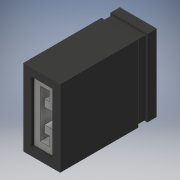
# Autodesk Inventor part: Jumper
Saved by Autodesk Inventor 2017 SP1 (Build 210196100, 196)
## iProperties
Part Number: Jumper
Material: Generisch
Document SubType Name: Modeling
Designer: Alex
Density: 1 g/cm^3
Appearance: Vorgabe
Author: Alex
Autodesk Inventor part; units mm, degrees
ref_plane "YZ Plane" through (0, 0, 0) normal (1, 0, 0) x (0, 1, 0)
ref_plane "XZ Plane" through (0, 0, 0) normal (0, 1, 0) x (-1, 0, 0)
sketch "Skizze2" plane through (0, 0, 0) normal (0, 1, 0) x (-1, 0, 0)
  line L0 (0, 0) -> (2.4, 0)
  line L1 (2.4, 0) -> (2.4, -5)
  line L2 (2.4, -5) -> (0, -5)
  line L3 (0, -5) -> (0, 0)
  dimension "d0" = 2.4
  dimension "d1" = 5
  constraints: 8 end point, 2 parallel, 1 coincident, 1 horizontal, 1 perpendicular
  measures "d0" distance of L1.end L2.end
  measures "d1" distance of L0.end L1.end
extrude "Extrusion1" add sketch "Skizze2" along normal blind 6.3
sketch "Skizze3" plane through (0, 0, 0) normal (0, -1, 0) x (1, 0, 0)
  line L0 (-0.9, -3.47) -> (-1.5, -3.47)
  line L1 (-1.5, -3.47) -> (-1.5, -4.07)
  line L2 (-1.5, -4.07) -> (-0.9, -4.07)
  line L3 (-0.9, -4.07) -> (-0.9, -3.47)
  line L4 (-0.9, -0.93) -> (-1.5, -0.93)
  line L5 (-1.5, -0.93) -> (-1.5, -1.53)
  line L6 (-1.5, -1.53) -> (-0.9, -1.53)
  line L7 (-0.9, -1.53) -> (-0.9, -0.93)
  line L8 (-2.4, -5) -> (0, -5) projected
  line L9 (-2.4, 0) -> (-2.4, -5) projected
  point P0 (0, 0)
  dimension "d4" = 0.6
  dimension "d5" = 0.6
  dimension "d6" = 0.6
  dimension "d7" = 0.6
  dimension "d8" = 2.54
  dimension "d9" = 0.93
  dimension "d10" = 0.9
  dimension "d11" = 0.9
  constraints: 16 end point, 4 parallel, 2 horizontal, 2 perpendicular
  measures "d4" distance of L1.end L2.end
  measures "d5" distance of L2.end L0.start
  measures "d6" distance of L6.end L4.start
  measures "d7" distance of L5.end L6.end
  measures "d8" distance between parallel lines of L2 L6
  measures "d9" distance between parallel lines of L8 L2
  measures "d10" distance between parallel lines of L9 L1
  measures "d11" distance between parallel lines of L9 L5
sketch "Skizze5" plane through (0, 0, 0) normal (0, -1, 0) x (1, 0, 0)
  line L0 (-0.5, -0.5) -> (-1.9, -0.5)
  line L1 (-1.9, -0.5) -> (-1.9, -4.5)
  line L2 (-1.9, -4.5) -> (-0.5, -4.5)
  line L3 (-0.5, -4.5) -> (-0.5, -0.5)
  line L4 (-2.4, 0) -> (-2.4, -5) projected
  line L5 (0, -5) -> (-2.4, -5) projected
  point P0 (0, 0)
  dimension "d15" = 1.4
  dimension "d16" = 4
  dimension "d17" = 0.5
  dimension "d18" = 0.5
  constraints: 8 end point, 2 parallel, 1 horizontal, 1 perpendicular
  measures "d15" distance of L2.end L1.end
  measures "d16" distance of L1.end L0.end
  measures "d17" distance between parallel lines of L4 L1
  measures "d18" distance between parallel lines of L5 L2
extrude "Extrusion2" cut sketch "Skizze5" against normal blind 0.2
extrude "Extrusion3" cut sketch "Skizze3" against normal blind 6
ref_plane "Arbeitsebene1" through (0, 5.7, 0) normal (0, 1, 0) x (1, 0, 0)
sketch "Skizze6" plane through (0, 5.7, 0) normal (0, 1, 0) x (1, 0, 0)
  line L0 (1, -1) -> (-3, -1)
  line L1 (-3, -1) -> (-3, 6)
  line L2 (-3, 6) -> (1, 6)
  line L3 (1, 6) -> (1, -1)
  line L4 (-0.1, 4.9) -> (-2.3, 4.9)
  line L5 (-2.3, 4.9) -> (-2.3, 0.1)
  line L6 (-2.3, 0.1) -> (-0.1, 0.1)
  line L7 (-0.1, 0.1) -> (-0.1, 4.9)
  line L8 (0, 5) -> (-2.4, 5) projected
  line L9 (0, 0) -> (0, 5) projected
  line L10 (0, 0) -> (-2.4, 0) projected
  line L11 (-2.4, 5) -> (-2.4, 0) projected
  dimension "d24" = 0.1
  dimension "d25" = 0.1
  dimension "d26" = 0.1
  dimension "d27" = 0.1
  constraints: 16 end point, 4 parallel, 2 horizontal, 2 perpendicular
  measures "d24" distance between parallel lines of L8 L4
  measures "d25" distance between parallel lines of L9 L7
  measures "d26" distance between parallel lines of L10 L6
  measures "d27" distance between parallel lines of L11 L5
extrude "Extrusion5" cut sketch "Skizze6" against normal blind 0.6 contours L0 L1 L2 L3 | L9 L10 L11 L8
sketch "Skizze7" plane through (0, 0.2, 0) normal (0, -1, 0) x (1, 0, 0)
  line L0 (-0.5, -2.004) -> (-1.5, -2.004)
  line L1 (-1.5, -2.004) -> (-1.5, -2.996)
  line L2 (-1.5, -2.996) -> (-0.5, -2.996)
  line L3 (-0.5, -2.996) -> (-0.5, -2.004)
  line L4 (-1.5, -3.47) -> (-0.9, -3.47) projected
  line L5 (-0.9, -1.53) -> (-1.5, -1.53) projected
  line L6 (-0.5, -0.5) -> (-0.5, -4.5) projected
  line L7 (-1.5, -1.53) -> (-1.5, -0.93) projected
  line L8 (-1.5, -2.004) -> (-1.217, -2.004)
  line L9 (-1.217, -2.004) -> (-1.217, -1.53)
  line L10 (-1.217, -1.53) -> (-1.5, -1.53)
  line L11 (-1.5, -1.53) -> (-1.5, -2.004)
  line L12 (-1.5, -3.47) -> (-0.9, -3.47) projected
  line L13 (-1.5, -2.996) -> (-1.217, -2.996)
  line L14 (-1.217, -2.996) -> (-1.217, -3.47)
  line L15 (-1.217, -3.47) -> (-1.5, -3.47)
  line L16 (-1.5, -3.47) -> (-1.5, -2.996)
  point P0 (0, 0)
  dimension "d32" = 0.474
  dimension "d33" = 0.474
  dimension "d34" = 0.283
  dimension "d35" = 0.283
  constraints: 24 end point, 6 parallel, 3 horizontal, 3 perpendicular, 2 collinear, 2 point on line
  measures "d32" distance between parallel lines of L2 L4
  measures "d33" distance between parallel lines of L5 L0
  measures "d34" distance of L10.end L9.end
  measures "d35" distance of L14.end L15.end
extrude "Extrusion6" cut sketch "Skizze7" against normal up to surface (5.8 mm away)
